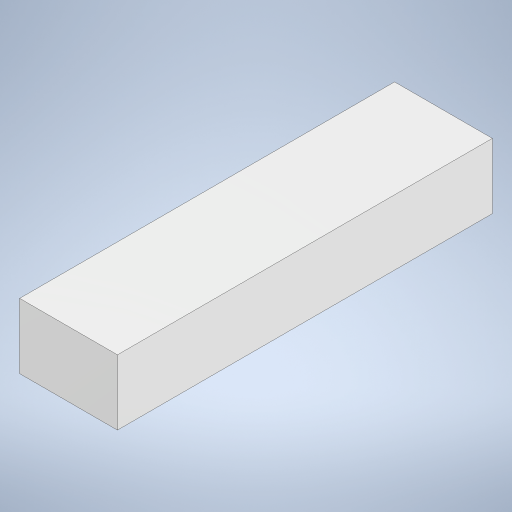
# Autodesk Inventor part: Batteryv2
Saved by Autodesk Inventor 2024 (Build 280153000, 153)
## iProperties
Created: 2024-03-09
Part Number: Batteryv2
Material: PC/ABS Plastic
Document SubType Name: Modeling
Designer: kdcao
Density: 1.1 g/cm^3
Appearance: Smooth - White
Author: kdcao
Autodesk Inventor part; units mm, degrees
ref_plane "YZ Plane" through (0, 0, 0) normal (1, 0, 0) x (0, 1, 0)
ref_plane "XZ Plane" through (0, 0, 0) normal (0, 1, 0) x (-1, 0, 0)
ref_plane "XY Plane" through (0, 0, 0) normal (0, 0, 1) x (1, 0, 0)
sketch "Sketch1" plane through (0, 0, 0) normal (0, 1, 0) x (-1, 0, 0)
  line L0 (-9, 34.5) -> (9, 34.5)
  line L1 (9, 34.5) -> (9, -34.5)
  line L2 (9, -34.5) -> (-9, -34.5)
  line L3 (-9, -34.5) -> (-9, 34.5)
  line L4 (-9, 34.5) -> (9, -34.5) construction
  line L5 (9, 34.5) -> (-9, -34.5) construction
  point P0 (0, 0)
  dimension "d0" = 69
  dimension "d1" = 18
  constraints: 12 end point, 2 midpoint, 2 parallel, 1 horizontal, 1 perpendicular
  measures "d0" distance of L0.end L1.end
  measures "d1" distance of L0.start L0.end
extrude "Extrusion1" add sketch "Sketch1" along normal blind 12
body "Solid1"
